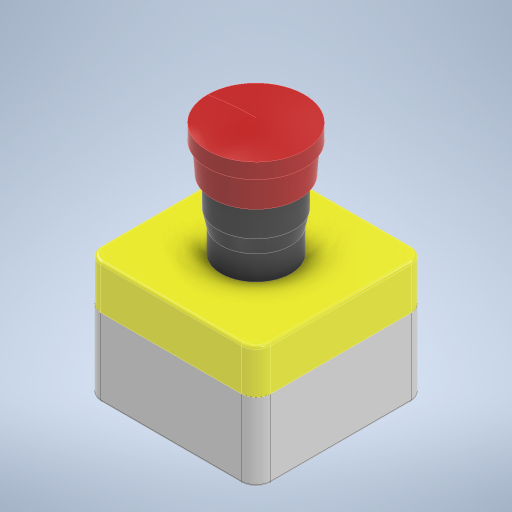
# Autodesk Inventor part: stop-button
Saved by Autodesk Inventor 2023 (Build 270158030, 158C)
## iProperties
Created: 2024-04-03
Part Number: stop-button
Material: Generic
Document SubType Name: Modeling
Designer: Imogen Heard
Density: 1 g/cm^3
Appearance: Default
Author: Imogen Heard
Autodesk Inventor part; units mm, degrees
ref_plane "YZ Plane" through (0, 0, 0) normal (1, 0, 0) x (0, 1, 0)
ref_plane "XZ Plane" through (0, 0, 0) normal (0, 1, 0) x (-1, 0, 0)
ref_plane "XY Plane" through (0, 0, 0) normal (0, 0, 1) x (1, 0, 0)
sketch "Sketch1" plane through (0, 0, 0) normal (0, 1, 0) x (-1, 0, 0)
  line L0 (34.825, -34.8) -> (-34.825, -34.8)
  line L1 (-34.825, -34.8) -> (-34.825, 34.8)
  line L2 (-34.825, 34.8) -> (34.825, 34.8)
  line L3 (34.825, 34.8) -> (34.825, -34.8)
  circle A0 centre (-17.825, -28.8) radius 2.3
  circle A1 centre (17.825, 28.8) radius 2.3
  point P0 (0, 0)
  dimension "d0" = 69.65
  dimension "d1" = 69.6
  dimension "d2" = 34.8
  dimension "d3" = 34.825
  dimension "d4" = 4.6
  dimension "d5" = 17
  dimension "d6" = 6
  dimension "d7" = 6
  dimension "d8" = 17
  constraints: 8 end point, 2 centre point, 2 parallel, 1 equal radius, 1 horizontal, 1 perpendicular
  measures "d0" distance between parallel lines of L1 L3
  measures "d1" distance between parallel lines of L2 L0
  measures "d2" distance from line of point (0, 0) L0
  measures "d3" distance from line of point (0, 0) L1
  measures "d4" diameter of A0
  measures "d5" distance from line of L1 A0.centre
  measures "d6" distance from line of L0 A0.centre
  measures "d7" distance from line of L2 A1.centre
  measures "d8" distance from line of L3 A1.centre
extrude "Extrusion1" add sketch "Sketch1" along normal blind 2.6
sketch "Sketch2" plane through (0, 2.6, 0) normal (0, 1, 0) x (1, 0, 0)
  line L0 (-34.825, -34.8) -> (34.825, -34.8) projected
  line L1 (34.825, -34.8) -> (34.825, 34.8) projected
  line L2 (34.825, 34.8) -> (-34.825, 34.8) projected
  line L3 (-34.825, 34.8) -> (-34.825, -34.8) projected
  circle A0 centre (-17.825, -28.8) radius 2.3 projected
  circle A1 centre (17.825, 28.8) radius 2.3 projected
  line L4 (-33.705, -33.68) -> (33.705, -33.68)
  line L5 (33.705, -33.68) -> (33.705, 33.68)
  line L6 (33.705, 33.68) -> (-33.705, 33.68)
  line L7 (-33.705, 33.68) -> (-33.705, -33.68)
  point P0 (0, 0)
  dimension "d11" = 1.12
  constraints: 8 end point, 3 other
  measures "d11" distance between parallel lines of L7 L3
extrude "Extrusion2" add sketch "Sketch2" along normal blind 29.4 contours L3 L2 L1 L0
fillet "Fillet1" radius 5 4 edges at (-33.705, 17.3, 33.68) (-33.705, 17.3, -33.68) (33.705, 17.3, -33.68) (33.705, 17.3, 33.68)
fillet "Fillet2" radius 6 4 edges at (-34.825, 16, -34.8) (34.825, 16, -34.8) (34.825, 16, 34.8) (-34.825, 16, 34.8)
fillet "Fillet3" radius 1 8 edges at (33.0676, 0, 33.0426) (34.825, 0, 0) (33.0676, 0, -33.0426) (0, 0, -34.8) (-33.0676, 0, -33.0426) (-34.825, 0, 0) (-33.0676, 0, 33.0426) (0, 0, 34.8)
sketch "Sketch3" plane through (0, 32, 0) normal (0, 1, 0) x (1, 0, 0)
  arc A0 (-34.825, -28.8) -> (-28.825, -34.8) centre (-28.825, -28.8) ccw projected
  line L0 (-28.825, -34.8) -> (28.825, -34.8) projected
  arc A1 (28.825, -34.8) -> (34.825, -28.8) centre (28.825, -28.8) ccw projected
  line L1 (34.825, -28.8) -> (34.825, 28.8) projected
  arc A2 (34.825, 28.8) -> (28.825, 34.8) centre (28.825, 28.8) ccw projected
  line L2 (28.825, 34.8) -> (-28.825, 34.8) projected
  arc A3 (-28.825, 34.8) -> (-34.825, 28.8) centre (-28.825, 28.8) ccw projected
  line L3 (-34.825, 28.8) -> (-34.825, -28.8) projected
  line L4 (-33.705, -28.68) -> (-33.705, 28.68) projected
  arc A4 (-28.705, 33.68) -> (-33.705, 28.68) centre (-28.705, 28.68) ccw projected
  line L5 (-28.705, 33.68) -> (28.705, 33.68) projected
  arc A5 (33.705, 28.68) -> (28.705, 33.68) centre (28.705, 28.68) ccw projected
  line L6 (33.705, 28.68) -> (33.705, -28.68) projected
  arc A6 (28.705, -33.68) -> (33.705, -28.68) centre (28.705, -28.68) ccw projected
  line L7 (28.705, -33.68) -> (-28.705, -33.68) projected
  arc A7 (-33.705, -28.68) -> (-28.705, -33.68) centre (-28.705, -28.68) ccw projected
  point P0 (0, 0)
extrude "Extrusion3" add sketch "Sketch3" along normal blind 18 separate body
sketch "Sketch4" plane through (0, 50, 0) normal (0, 1, 0) x (1, 0, 0)
  line L0 (-28.825, -34.8) -> (28.825, -34.8) projected
  arc A0 (28.825, -34.8) -> (34.825, -28.8) centre (28.825, -28.8) ccw projected
  line L1 (34.825, -28.8) -> (34.825, 28.8) projected
  arc A1 (34.825, 28.8) -> (28.825, 34.8) centre (28.825, 28.8) ccw projected
  line L2 (28.825, 34.8) -> (-28.825, 34.8) projected
  arc A2 (-28.825, 34.8) -> (-34.825, 28.8) centre (-28.825, 28.8) ccw projected
  line L3 (-34.825, 28.8) -> (-34.825, -28.8) projected
  arc A3 (-34.825, -28.8) -> (-28.825, -34.8) centre (-28.825, -28.8) ccw projected
  line L4 (28.705, -33.68) -> (-28.705, -33.68) projected
  arc A4 (-33.705, -28.68) -> (-28.705, -33.68) centre (-28.705, -28.68) ccw projected
  line L5 (-33.705, -28.68) -> (-33.705, 28.68) projected
  arc A5 (-28.705, 33.68) -> (-33.705, 28.68) centre (-28.705, 28.68) ccw projected
  line L6 (-28.705, 33.68) -> (28.705, 33.68) projected
  arc A6 (33.705, 28.68) -> (28.705, 33.68) centre (28.705, 28.68) ccw projected
  line L7 (33.705, 28.68) -> (33.705, -28.68) projected
  arc A7 (28.705, -33.68) -> (33.705, -28.68) centre (28.705, -28.68) ccw projected
  point P0 (0, 0)
extrude "Extrusion4" add sketch "Sketch4" against normal blind 1.1 contours L4 A4 L5 A5 L6 A6 L7 A7 bodies 2
fillet "Fillet4" radius 1 8 edges at (33.0676, 50, 33.0426) (34.825, 50, 0) (33.0676, 50, -33.0426) (0, 50, -34.8) (-33.0676, 50, -33.0426) (-34.825, 50, 0) (-33.0676, 50, 33.0426) (0, 50, 34.8)
sketch "Sketch5" plane through (0, 50, 0) normal (0, 1, 0) x (1, 0, 0)
  circle A0 centre (0, 0) radius 14.3
  dimension "d22" = 28.6
  constraints: 1 centre point, 1 coincident
  measures "d22" diameter of A0
extrude "Extrusion5" add sketch "Sketch5" along normal blind 10 separate body
sketch "Sketch6" plane through (0, 60, 0) normal (0, 1, 0) x (1, 0, 0)
  circle A0 centre (0, 0) radius 14.3 projected
extrude "Extrusion6" add sketch "Sketch6" along normal blind 6.26 draft 12 bodies 3
sketch "Sketch7" plane through (0, 66.26, 0) normal (0, 1, 0) x (1, 0, 0)
  circle A0 centre (0, 0) radius 15.6306 projected
extrude "Extrusion7" add sketch "Sketch7" along normal blind 12 bodies 3
sketch "Sketch8" plane through (0, 78.26, 0) normal (0, 1, 0) x (1, 0, 0)
  circle A0 centre (0, 0) radius 15.6306 projected
  circle A1 centre (0, 0) radius 17.75
  dimension "d29" = 35.5
  constraints: 1 centre point, 1 coincident
  measures "d29" diameter of A1
extrude "Extrusion8" add sketch "Sketch8" along normal blind 12 draft 4 separate body contours A0 | A1
sketch "Sketch10" plane through (0, 0, 0) normal (0, 0, 1) x (1, 0, 0)
  line L0 (-18.5891, 90.26) -> (18.5891, 90.26) projected
  line L1 (0, 90.26) -> (-19.85, 90.26)
  line L2 (-19.85, 90.26) -> (-19.85, 96.52)
  line L3 (-19.85, 96.52) -> (0, 96.52)
  line L4 (0, 96.52) -> (0, 90.26)
  line L5 (-19.85, 96.52) -> (-9, 98.26) construction
  line L6 (-9, 98.26) -> (0, 98.26) construction
  spline S0 degree 2 poles (-19.85, 96.52) (-9, 98.26) (0, 98.26) knots 1 1 1 2 2 2
  line L7 (0, 98.26) -> (0, 96.52)
  point P0 (0, 0)
  dimension "d35" = 19.85
  dimension "d36" = 6.26
  dimension "d37" = 8
  dimension "d38" = 9
  constraints: 10 end point, 3 parallel, 1 horizontal, 1 midpoint, 1 perpendicular, 1 vertical, 3 other
  measures "d35" distance between parallel lines of L4 L2
  measures "d36" distance between parallel lines of L0 L3
  measures "d37" distance from line of L0 L6.end
  measures "d38" distance from line of L4 L5.end
revolve "Revolution1" add sketch "Sketch10" angle 360 about axis through (0, 96.52, 0) along (0, -1, 0) bodies 4
sketch "Sketch11" plane through (0, 2.6, 0) normal (0, 1, 0) x (1, 0, 0)
  circle A0 centre (19.825, 0) radius 9.5
  circle A1 centre (-19.825, 0) radius 9.5
  line L0 (-34.825, 28.8) -> (-34.825, -28.8) projected
  line L1 (34.825, -28.8) -> (34.825, 28.8) projected
  line L2 (33.705, 28.68) -> (33.705, -28.68) projected
  point P0 (0, 0)
  point P1 (33.705, 0)
  dimension "d40" = 19
  dimension "d41" = 15
  dimension "d42" = 15
  constraints: 2 centre point, 2 horizontal alignment, 1 equal radius, 1 midpoint
  measures "d40" diameter of A1
  measures "d41" distance from line of L0 A1.centre
  measures "d42" distance from line of L1 A0.centre
extrude "Extrusion10" cut sketch "Sketch11" against normal blind 1 bodies 1
sketch "Sketch9" plane through (0, 90.26, 0) normal (0, 1, 0) x (1, 0, 0)
  circle A0 centre (0, 0) radius 19.8
  dimension "d32" = 39.6
  constraints: 1 centre point, 1 coincident
  measures "d32" diameter of A0
equation "\"d2\" = 0.5 * d1"
equation "\"d3\" = 0.5 * d0"
body "Solid1"
